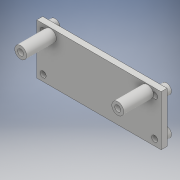
# Autodesk Inventor part: Soporte 16 pwm
Saved by Autodesk Inventor 2018 (Build 220112000, 112)
## iProperties
Created: 2018-03-08
Part Number: Soporte 16 pwm
Material: Genérico
Document SubType Name: Modeling
Designer: ivanb
Density: 1 g/cm^3
Appearance: Valor por defecto
Author: ivanb
Autodesk Inventor part; units mm, degrees
ref_plane "YZ Plane" through (0, 0, 0) normal (1, 0, 0) x (0, 1, 0)
ref_plane "XZ Plane" through (0, 0, 0) normal (0, 1, 0) x (-1, 0, 0)
ref_plane "XY Plane" through (0, 0, 0) normal (0, 0, 1) x (1, 0, 0)
sketch "Boceto1" plane through (0, 0, 0) normal (0, 1, 0) x (-1, 0, 0)
  circle A0 centre (22.76, 7.95) radius 1.5
  circle A1 centre (-26.24, 7.95) radius 1.5
  line L0 (29.635, -14.19) -> (29.635, 11.2)
  line L1 (29.635, 11.2) -> (-33.115, 11.2)
  line L2 (-33.115, 11.2) -> (-33.115, -14.19)
  line L3 (-33.115, -14.19) -> (29.635, -14.19)
  line L4 (-1.74, -3.0983) -> (-1.74, -1.495)
  line L5 (-1.74, -1.495) -> (-3.5727, -1.495)
  circle A2 centre (26.385, -10.94) radius 1.5
  circle A3 centre (-29.865, -10.94) radius 1.5
  circle A4 centre (26.385, 7.95) radius 1.5
  circle A5 centre (-29.865, 7.95) radius 1.5
  dimension "d5" = 25.39
  dimension "d6" = 62.75
  dimension "d7" = 3
  dimension "d8" = 3.25
  dimension "d9" = 3.25
  dimension "d10" = 49
  dimension "d11" = 0
  dimension "d24" = 3
  constraints: 12 end point, 6 centre point, 4 symmetric about line, 3 coincident, 2 parallel, 2 perpendicular, 6 other
  measures "d5" distance of L2.end L1.end
  measures "d6" distance of L1.end L0.end
  measures "d7" diameter of A2
  measures "d8" distance from line of L3 A2.centre
  measures "d9" distance from line of L0 A2.centre
  measures "d10" distance of A1.centre A0.centre
  measures "d11" vertical distance of A4.centre A0.centre
  measures "d24" diameter of A0
extrude "Extrusión1" add sketch "Boceto1" along normal blind 3
sketch "Boceto2" plane through (0, 3, 0) normal (0, 1, 0) x (1, 0, 0)
  circle A0 centre (-26.385, -7.95) radius 1.5 projected
  circle A1 centre (-26.385, -7.95) radius 2.5
  circle A2 centre (-26.385, 10.94) radius 1.5 projected
  circle A3 centre (-26.385, 10.94) radius 2.5
  circle A4 centre (29.865, 10.94) radius 1.5 projected
  circle A5 centre (29.865, 10.94) radius 2.5
  circle A6 centre (29.865, -7.95) radius 1.5 projected
  circle A7 centre (29.865, -7.95) radius 2.5
  point P0 (0, 0)
  dimension "d14" = 5
  dimension "d15" = 5
  dimension "d16" = 5
  dimension "d17" = 5
  constraints: 4 centre point, 4 coincident
  measures "d14" diameter of A1
  measures "d15" diameter of A3
  measures "d16" diameter of A5
  measures "d17" diameter of A7
extrude "Extrusión2" add sketch "Boceto2" along normal blind 3
sketch "Boceto3" plane through (0, 0, 0) normal (0, -1, 0) x (1, 0, 0)
  circle A0 centre (-22.76, 7.95) radius 1.5 projected
  circle A1 centre (-22.76, 7.95) radius 3
  circle A2 centre (26.24, 7.95) radius 1.5 projected
  circle A3 centre (26.24, 7.95) radius 3
  point P0 (0, 0)
  dimension "d20" = 6
  dimension "d21" = 6
  constraints: 2 centre point, 2 coincident
  measures "d20" diameter of A1
  measures "d21" diameter of A3
extrude "Extrusión3" add sketch "Boceto3" along normal blind 15
